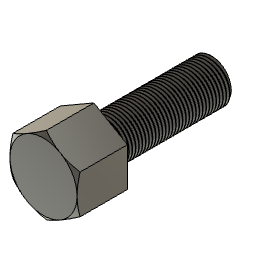
03 (Autodesk Fusion 360 design; units mm, degrees)
Autodesk Fusion 360 part; units mm, degrees
sketch "Sketch1" plane through (0, 0, 0) normal (0, 1, 0) x (1, 0, 0)
  line L0 (20, 11.547) -> (0, 23.094)
  line L1 (0, 23.094) -> (-20, 11.547)
  line L2 (-20, 11.547) -> (-20, -11.547)
  line L3 (-20, -11.547) -> (0, -23.094)
  line L4 (0, -23.094) -> (20, -11.547)
  line L5 (20, -11.547) -> (20, 11.547)
extrude "Extrude1" add sketch "Sketch1" along normal blind 30
sketch "Sketch2" plane through (0, 0, 0) normal (0, -1, 0) x (1, 0, 0)
  circle A0 centre (0, 0) radius 20
  line L0 (20, 11.547) -> (20, -11.547)
  constraint coincident A0.centre origin
  constraint tangent A0 L0
extrude "Extrude2" cut sketch "Sketch2" against normal through all draft 60 keep common part
sketch "Sketch3" plane through (0, 30, 0) normal (0, 1, 0) x (-1, 0, 0)
  circle A0 centre (0, 0) radius 12.5
  dimension "d4" = 25
  constraint coincident A0.centre origin
  measures "d4" diameter of A0
extrude "Extrude3" add sketch "Sketch3" along normal blind 70
thread "Thread2" "ISO Metric profile 25.0 M25x2 6g" major diameter 24.822 minor diameter 22.5289 pitch 2 angle 60 modelled right hand crest width 0.2818 on face at (-12.4379, 76.6667, -1.2446) crest through (-12.411, 29.5, 0)
thread "Thread1" [suppressed]
